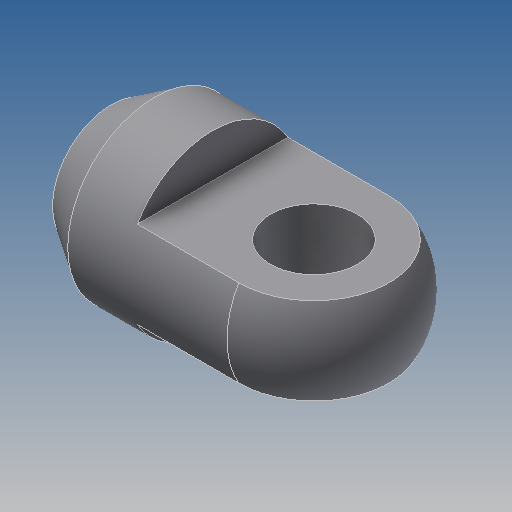
# Autodesk Inventor part: Stangenkopf
Saved by Autodesk Inventor 2018 (Build 220112000, 112)
## iProperties
Created: 2018-10-20
Part Number: Stangenkopf
Material: Generisch
Document SubType Name: Modeling
Designer: M.Knabel
Density: 1 g/cm^3
Appearance: Vorgabe
Mass: 0.144452 g
Surface Area: 2.43562 cm^2
Volume: 0.144452 cm^3
Author: M.Knabel
Autodesk Inventor part; units mm, degrees
ref_plane "YZ Plane" through (0, 0, 0) normal (1, 0, 0) x (0, 1, 0)
ref_plane "XY Plane" through (0, 0, 0) normal (0, 0, 1) x (1, 0, 0)
sketch "Skizze1" plane through (0, 0, 0) normal (0, 0, 1) x (1, 0, 0)
  line L0 (0, -0.6) -> (0, 3.6) projected
  line L1 (-2, 0) -> (12, 0) projected
  line L2 (0, 0) -> (10, 0)
  line L3 (10, 0) -> (10, 3)
  line L4 (10, 3) -> (0, 3)
  line L5 (0, 3) -> (0, 0)
  dimension "d1" = 10
  dimension "d2" = 6
  constraints: 8 end point, 2 parallel, 1 horizontal, 1 perpendicular
  measures "d1" distance between parallel lines of L3 L0
  measures "d2" diameter of L4 L1
revolve "Umdrehung1" add sketch "Skizze1" angle 360 about axis through (-10, 0, 0) along (1, 0, 0)
ref_plane "Arbeitsebene1" through (5, -3, 0) normal (0, 1, 0) x (-1, 0, 0)
sketch "Skizze2" plane through (5, -3, 0) normal (0, 1, 0) x (-1, 0, 0)
  line L0 (5, 3) -> (5, -3) projected
  line L1 (-5, 3) -> (-5, -3) projected
  line L2 (5, -3) -> (-5, -3) projected
  line L3 (5, 3) -> (-5, 3) projected
  line L4 (1.5, 3) -> (1.5, 1.5)
  line L5 (1.5, 1.5) -> (-5, 1.5)
  line L6 (-5, -1.5) -> (1.5, -1.5)
  line L7 (1.5, -1.5) -> (1.5, -3)
  line L8 (-5, 1.5) -> (-5, 3)
  line L9 (-5, 3) -> (1.5, 3)
  line L10 (-5, 3) -> (-5, -3) projected
  line L11 (-5, -1.5) -> (-5, -3)
  line L12 (-5, -3) -> (1.5, -3)
  dimension "d4" = 1.5
  dimension "d5" = 1.5
  dimension "d6" = 3.5
  constraints: 16 end point, 4 perpendicular, 3 collinear, 3 point on line
  measures "d4" distance between parallel lines of L3 L5
  measures "d5" distance between parallel lines of L2 L6
  measures "d6" distance between parallel lines of L0 L4
extrude "Extrusion1" cut sketch "Skizze2" along normal through all contours L4 L5 L1 L3 | L2 L1 L6 L7
chamfer "Fase1" distance 1.5 angle 33 1 edges at (0, -3, 0) measured on face at (4.5, -2.8079, -1.0563)
sketch "Skizze3" plane through (3.5, 2.5981, 1.5) normal (0, 0, 1) x (1, 0, 0)
  line L0 (6.5, 0) -> (6.5, -5.1962) construction
  arc A0 (3.5, -5.5981) -> (3.5, 0.4019) centre (3.5, -2.5981) ccw
  line L1 (6.5, 0) -> (6.5, 0.4019) projected
  line L2 (3.5, 0.4019) -> (7.092, 0.4019)
  line L3 (-2, 0.4019) -> (6.5, 0.4019) projected
  line L4 (7.092, 0.4019) -> (7.092, -5.5981)
  line L5 (7.092, -5.5981) -> (3.5, -5.5981)
  line L6 (-5.6184, -5.5981) -> (9.2105, -5.5981) projected
  point P0 (-3.5, -2.5981)
  point P1 (6.5, -5.5981)
  dimension "d13" = 3
  dimension "d14" = 3.592
  constraints: 6 end point, 3 collinear, 2 perpendicular, 2 point on circle, 2 tangent, 1 centre point
  measures "d13" distance from line of A0.centre L0
  measures "d14" distance from line of A0.centre L4
extrude "Extrusion2" cut sketch "Skizze3" against normal through all
sketch "Skizze4" plane through (3.5, -2.5981, 1.5) normal (0, 0, 1) x (1, 0, 0)
  arc A0 (5, 0) -> (5, 5.1962) centre (3.5, 2.5981) ccw projected
  point P0 (-3.5, 2.5981)
  constraints: 1 coincident
hole "Bohrung1" at (7, 0, 1.5) at (7, 0, 1.5) direction (0, 0, -1) diameter 3 depth 3 tip angle 118
sketch "Skizze7" plane through (0, 0, 0) normal (-1, 0, 0) x (0, 0, 1)
  arc A0 (1.5, 2.5981) -> (-1.5, 2.5981) centre (0, 0) ccw
  circle A1 centre (0, 0) radius 3 construction
  line L0 (-1.5, 2.5981) -> (-1.5, 4)
  line L1 (-1.5, 4) -> (1.5, 4)
  line L2 (1.5, 4) -> (1.5, 2.5981)
  line L3 (0, -4.5424) -> (0, 5.5632) projected
  dimension "d25" = 1.5
  dimension "d26" = 3
  dimension "d27" = 4
  constraints: 6 end point, 4 point on circle, 2 perpendicular, 1 centre point, 1 coincident, 1 vertical
  measures "d25" distance between parallel lines of L3 L0
  measures "d26" distance between parallel lines of L2 L0
  measures "d27" distance from line of point (0, 0) L1
sketch "Skizze8" plane through (3.5, -2.5981, 1.5) normal (0, 0, 1) x (1, 0, 0)
  line L0 (-2, 5.5981) -> (3.5, 5.5981) projected
  line L1 (3.5, 5.5981) -> (-3.5, 5.5981)
  arc A0 (5, 0) -> (5, 5.1962) centre (3.5, 2.5981) ccw projected
  arc A1 (3.5, -0.4019) -> (3.5, 5.5981) centre (3.5, 2.5981) ccw
  line L2 (-2, -0.4019) -> (3.5, -0.4019) projected
  line L3 (3.5, -0.4019) -> (-2.8962, -0.4019)
  point P0 (-3.5, 2.5981)
  constraints: 4 end point, 2 collinear, 2 point on circle, 2 point on line, 1 centre point, 1 coincident, 1 tangent
sweep "Sweeping2" cut profiles "Skizze7" path "Skizze8" path curves L1 A1 L3
sketch "Skizze9" plane through (0, 0, 0) normal (-1, 0, 0) x (0, 0, 1)
  point P0 (0, 0)
  point P1 (0, 0)
  constraints: 1 coincident
hole "Bohrung2" at (0, 0, 0) direction (1, 0, 0) diameter 2.459 depth 4 tip angle 118
